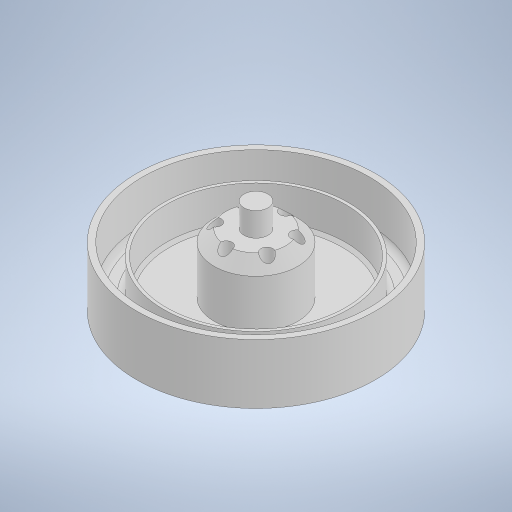
# Autodesk Inventor part: Wheel Mold
Saved by Autodesk Inventor 2023.2 (Build 272271000, 271)
## iProperties
Created: 2023-03-10
Part Number: Wheel Mold
Material: Generic
Document SubType Name: Modeling
Designer: Nathan Cai
Density: 1 g/cm^3
Appearance: Default
Author: Nathan Cai
Autodesk Inventor part; units mm, degrees
ref_plane "YZ Plane" through (0, 0, 0) normal (1, 0, 0) x (0, 1, 0)
ref_plane "XZ Plane" through (0, 0, 0) normal (0, 1, 0) x (-1, 0, 0)
ref_plane "XY Plane" through (0, 0, 0) normal (0, 0, 1) x (1, 0, 0)
sketch "Sketch1" plane through (0, 0, 0) normal (0, 1, 0) x (-1, 0, 0)
  point P0 (0, 0)
sketch "Sketch2" plane through (0, 0, 0) normal (0, 1, 0) x (-1, 0, 0)
  circle A0 centre (0, 0) radius 31.75
  dimension "d0" = 63.5
  constraints: 1 centre point, 1 coincident
  measures "d0" diameter of A0
extrude "Extrusion1" add sketch "Sketch2" along normal blind 15.875
sketch "Sketch3" plane through (0, 15.875, 0) normal (0, 1, 0) x (1, 0, 0)
  circle A0 centre (0, 0) radius 23.8125
  dimension "d3" = 47.625
  constraints: 1 centre point, 1 coincident
  measures "d3" diameter of A0
extrude "Extrusion2" cut sketch "Sketch3" against normal blind 12.7
chamfer "Chamfer1" distance 0.7937 angle 45 1 edges at (-23.8125, 3.175, 0)
sketch "Sketch4" plane through (0, 3.175, 0) normal (0, 1, 0) x (1, 0, 0)
  circle A0 centre (0, 0) radius 11.1125
  dimension "d12" = 22.225
  constraints: 1 centre point, 1 coincident
  measures "d12" diameter of A0
extrude "Extrusion3" add sketch "Sketch4" along normal blind 15.875
sketch "Sketch5" plane through (0, 19.05, 0) normal (0, 1, 0) x (1, 0, 0)
  circle A0 centre (0, 0) radius 3.175
  dimension "d15" = 6.35
  constraints: 1 centre point, 1 coincident
  measures "d15" diameter of A0
extrude "Extrusion4" add sketch "Sketch5" along normal blind 6.35
chamfer "Chamfer3" distance 3.175 angle 45 1 edges at (-11.1125, 19.05, 0)
sketch "Sketch6" plane through (0, 19.05, 0) normal (0, 1, 0) x (1, 0, 0)
  circle A0 centre (0, 0) radius 7.9375 construction
  circle A1 centre (0, 0) radius 7.9375 projected
  circle A2 centre (0, 7.9375) radius 1.5875
  line L0 (0, 0) -> (0, 7.9375) construction
  circle A3 centre (-6.8741, 3.9688) radius 1.5875
  circle A4 centre (-6.8741, -3.9687) radius 1.5875
  circle A5 centre (0, -7.9375) radius 1.5875
  circle A6 centre (6.8741, -3.9688) radius 1.5875
  circle A7 centre (6.8741, 3.9687) radius 1.5875
  dimension "d21" = 15.875
  dimension "d22" = 3.175
  dimension "d25" = 360
  constraints: 7 centre point, 2 end point, 1 coincident, 1 vertical, 1 vertical alignment, 14 other
  measures "d21" diameter of A0
  measures "d22" diameter of A2
extrude "Extrusion5" cut sketch "Sketch6" against normal through all contours A7 A1 | A1 A7 | A6 A1 | A1 A6 | A2 A1 | A1 A2 | A5 A1 | A1 A5 | A3 A1 | A1 A3 | A4 A1 | A1 A4
sketch "Sketch8" plane through (0, 15.875, 0) normal (0, 1, 0) x (1, 0, 0)
  circle A0 centre (0, 0) radius 23.8125
  circle A1 centre (0, 0) radius 24.6063
  circle A2 centre (0, 0) radius 23.8125 projected
  circle A3 centre (0, 0) radius 31.75 projected
  circle A4 centre (0, 0) radius 3.175 projected
  circle A5 centre (0, 0) radius 30.1625
  dimension "d38" = 0.7937
  dimension "d39" = 47.625
  dimension "d40" = 1.5875
  constraints: 3 centre point, 3 coincident
  measures "d38" radial gap between concentric circles of A0 A1
  measures "d39" diameter of A0
  measures "d40" radial gap between concentric circles of A3 A5
extrude "Extrusion7" cut sketch "Sketch8" against normal blind 12.7 contours A5
fillet "Fillet1" radius 1.5875 2 edges at (-24.6063, 3.175, 0) (-30.1625, 3.175, 0)
sketch "Sketch9" plane through (0, 15.875, 0) normal (0, 1, 0) x (1, 0, 0)
  circle A0 centre (0, 0) radius 19.05
  circle A1 centre (0, 0) radius 25.4
  dimension "d44" = 38.1
  dimension "d45" = 50.8
  constraints: 2 centre point, 2 coincident
  measures "d44" diameter of A0
  measures "d45" diameter of A1
extrude "Extrusion8" cut sketch "Sketch9" against normal blind 3.175
body "Solid1"
